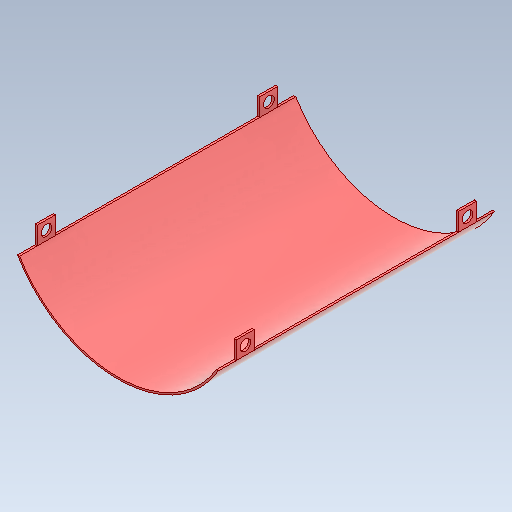
# Autodesk Inventor part: Obudowa, większa
Saved by Autodesk Inventor 2020 (Build 240168000, 168)
## iProperties
Created: 2021-10-14
Part Number: Obudowa, większa
Material: Ogólny
Document SubType Name: Modeling
Designer: Komputer
Density: 1 g/cm^3
Appearance: Gładkie — czerwone
Mass: 2.60871 g
Surface Area: 106.128 cm^2
Volume: 2.60871 cm^3
Author: Komputer
Autodesk Inventor part; units mm, degrees
ref_plane "YZ Plane" through (0, 0, 0) normal (1, 0, 0) x (0, 1, 0)
ref_plane "XZ Plane" through (0, 0, 0) normal (0, 1, 0) x (-1, 0, 0)
ref_plane "XY Plane" through (0, 0, 0) normal (0, 0, 1) x (1, 0, 0)
sketch "Szkic1" plane through (0, 0, 0) normal (0, 0, 1) x (1, 0, 0)
  circle A0 centre (0, 0) radius 32.5
  circle A1 centre (0, 0) radius 32
  dimension "d0" = 65
  dimension "d1" = 64
  constraints: 2 centre point, 2 coincident
  measures "d0" diameter of A0
  measures "d1" diameter of A1
extrude "Wyciągnięcie proste1" add sketch "Szkic1" along normal blind 77
sketch "Szkic2" plane through (0, 0, 77) normal (0, 0, 1) x (1, 0, 0)
  line L0 (0, 0) -> (-28, 0)
  line L1 (-28, 0) -> (-28, 15.4919)
  circle A0 centre (0, 0) radius 32 projected
  line L2 (-28, 0) -> (-28, -16.5)
  circle A1 centre (0, 0) radius 32.5 projected
  line L3 (-28, -16.5) -> (28, -16.5)
  line L4 (52.8927, -0.6882) -> (26.703, 44.9724)
  line L5 (26.703, 44.9724) -> (-31.7097, 42.3671)
  line L6 (-31.7097, 42.3671) -> (-48.5067, -13.9887)
  line L7 (-48.5067, -13.9887) -> (-28, -16.5)
  line L8 (28, -16.5) -> (52.8927, -0.6882)
  dimension "d4" = 28
  constraints: 18 end point, 2 horizontal, 2 point on circle, 1 perpendicular, 1 point on line, 2 other
  measures "d4" distance of L0.start L0.end
extrude "Wyciągnięcie proste2" cut sketch "Szkic2" against normal blind 77 contours L2 A0 L1 | L1 A0 L3 L2 | A0 L2 A1 L3 | A0 L3 L2 | L7 L6 L5 L4 L8 A1
sketch "Szkic3" plane through (-27.4181, -16.5, 77) normal (0, 1, 0) x (1, 0, 0)
  line L0 (-0.5819, 0) -> (55.4181, 0) projected
  line L1 (-0.5819, 0) -> (-0.5819, 5)
  line L2 (-0.5819, 0) -> (-0.5819, 77) projected
  line L3 (-0.5819, 5) -> (0, 5)
  line L4 (0, 77) -> (0, 0) projected
  line L5 (0, 5) -> (0, 10)
  line L6 (0, 10) -> (-0.5819, 10)
  line L7 (-0.5819, 10) -> (-0.5819, 5)
  line L8 (-0.5819, 77) -> (55.4181, 77) projected
  line L9 (-0.5819, 77) -> (-0.5819, 72)
  line L10 (-0.5819, 72) -> (0, 72)
  line L11 (0, 72) -> (0, 67)
  line L12 (0, 67) -> (-0.5819, 67)
  line L13 (-0.5819, 67) -> (-0.5819, 72)
  line L14 (55.4181, 77) -> (55.4181, 72)
  line L15 (55.4181, 77) -> (55.4181, 0) projected
  line L16 (55.4181, 72) -> (54.8361, 72)
  line L17 (54.8361, 0) -> (54.8361, 77) projected
  line L18 (54.8361, 72) -> (54.8361, 67)
  line L19 (54.8361, 67) -> (55.4181, 67)
  line L20 (55.4181, 67) -> (55.4181, 72)
  line L21 (55.4181, 0) -> (55.4181, 5)
  line L22 (55.4181, 5) -> (54.8361, 5)
  line L23 (54.8361, 5) -> (54.8361, 10)
  line L24 (54.8361, 10) -> (55.4181, 10)
  line L25 (55.4181, 10) -> (55.4181, 5)
  point P0 (27.4181, 77)
  dimension "d7" = 5
  dimension "d8" = 5
  dimension "d9" = 5
  dimension "d10" = 5
  dimension "d11" = 5
  dimension "d12" = 5
  dimension "d13" = 5
  dimension "d14" = 5
  constraints: 40 end point, 14 point on line, 10 perpendicular, 4 collinear
  measures "d7" distance of L0.start L1.end
  measures "d8" distance of L3.end L5.end
  measures "d9" distance of L2.end L9.end
  measures "d10" distance of L10.end L11.end
  measures "d11" distance of L8.end L14.end
  measures "d12" distance of L16.end L18.end
  measures "d13" distance of L0.end L21.end
  measures "d14" distance of L22.end L23.end
extrude "Wyciągnięcie proste3" add sketch "Szkic3" along normal blind 5 contours L2 L6 L4 L3 | L17 L24 L15 L22 | L2 L10 L4 L12 | L17 L16 L15 L19
sketch "Szkic4" plane through (28, -16.5, 67) normal (1, 0, 0) x (0, 0, -1)
  line L0 (57, 0) -> (57, 5) projected
  line L1 (62, 0) -> (62, 5) projected
  line L2 (57, 0) -> (62, 5)
  line L3 (62, 5) -> (57, 5) projected
  line L4 (62, 5) -> (57, 5)
  line L5 (57, 5) -> (62, 0)
  line L6 (0, 0) -> (-5, 0) projected
  line L7 (-5, 5) -> (0, 5) projected
  line L8 (-5, 0) -> (0, 5)
  line L9 (0, 5) -> (-5, 5)
  line L10 (-5, 5) -> (0, 0)
  circle A0 centre (-2.5, 2.5) radius 1.5
  circle A1 centre (59.5, 2.5) radius 1.5
  point P0 (67, 16.5)
  dimension "d17" = 3
  dimension "d18" = 3
  constraints: 12 end point, 2 centre point, 2 midpoint, 2 perpendicular, 1 collinear, 1 horizontal
  measures "d17" diameter of A0
  measures "d18" diameter of A1
extrude "Wyciągnięcie proste4" cut sketch "Szkic4" against normal up to surface (56 mm away) contours A1 L5 L2 | L2 L5 A1 | A1 L2 L5 | L2 A1 L5 | A0 L8 L10 | L10 L8 A0 | A0 L10 L8 | L10 A0 L8
